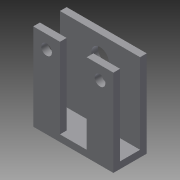
# Autodesk Inventor part: Speaker Mount
Saved by Autodesk Inventor 2014 SP2 (Build 180246200, 246)
## iProperties
Created: 2015-08-11
Part Number: Speaker Mount
Material: Generic
Document SubType Name: Modeling
Designer: Devon
Density: 1 g/cm^3
Appearance: Default
Author: Devon
Autodesk Inventor part; units mm, degrees
ref_plane "YZ Plane" through (0, 0, 0) normal (1, 0, 0) x (0, 1, 0)
ref_plane "XZ Plane" through (0, 0, 0) normal (0, 1, 0) x (-1, 0, 0)
ref_plane "XY Plane" through (0, 0, 0) normal (0, 0, 1) x (1, 0, 0)
sketch "Sketch1" plane through (0, 0, 0) normal (0, 0, 1) x (1, 0, 0)
  line L0 (-7.6264, 7.0378) -> (30.4736, 7.0378)
  line L1 (30.4736, 7.0378) -> (30.4736, -31.0622)
  line L2 (-7.6264, -31.0622) -> (-7.6264, 7.0378)
  circle A0 centre (11.4236, -2.4872) radius 4.1656
  circle A1 centre (11.4236, -21.5372) radius 4.1656
  line L3 (30.4736, -31.0622) -> (30.4736, -34.2372)
  line L4 (30.4736, -34.2372) -> (-7.6264, -34.2372)
  line L5 (-7.6264, -34.2372) -> (-7.6264, -31.0622)
  point P0 (0, 0)
  dimension "d0" = 38.1
  dimension "d1" = 38.1
  dimension "d4" = 8.3312
  dimension "d5" = 8.3312
  dimension "d8" = 3.175
  constraints: 12 end point, 2 centre point, 2 parallel, 2 perpendicular, 1 horizontal
  measures "d0" distance of L1.end L2.start
  measures "d1" distance of L0.end L1.end
  measures "d4" diameter of A0
  measures "d5" diameter of A1
  measures "d8" distance of L1.end L3.end
extrude "Extrusion1" add sketch "Sketch1" along normal blind 3.175
sketch "Sketch2" plane through (0, 0, 3.175) normal (0, 0, 1) x (1, 0, 0)
  line L0 (30.4736, -34.2372) -> (30.4736, 7.0378) projected
  line L1 (-7.6264, -34.2372) -> (30.4736, -34.2372)
  line L2 (30.4736, -34.2372) -> (30.4736, -31.0622)
  line L3 (30.4736, -31.0622) -> (-7.6264, -31.0622)
  line L4 (-7.6264, -31.0622) -> (-7.6264, -34.2372)
  point P0 (0, 0)
  dimension "d9" = 3.175
  constraints: 8 end point, 2 parallel, 1 horizontal, 1 perpendicular, 1 point on line
  measures "d9" distance of L2.end L1.end
extrude "Extrusion2" add sketch "Sketch2" along normal blind 12.7
sketch "Sketch3" plane through (-7.6264, -31.0622, 3.175) normal (0, 1, 0) x (1, 0, 0)
  line L0 (38.1, 0) -> (38.1, -12.7) projected
  line L1 (38.1, -12.7) -> (38.1, -9.525)
  line L2 (0, -9.525) -> (0, -12.7)
  line L3 (0, -9.525) -> (12.7, -9.525)
  line L4 (38.1, -9.525) -> (25.4, -9.525)
  line L5 (12.7, -9.525) -> (12.7, -12.7)
  line L6 (25.4, -9.525) -> (25.4, -12.7)
  line L7 (0, -12.7) -> (12.7, -12.7)
  line L8 (25.4, -12.7) -> (38.1, -12.7)
  point P0 (7.6264, 3.175)
  dimension "d12" = 3.175
  dimension "d13" = 12.7
  dimension "d14" = 12.7
  constraints: 16 end point, 5 perpendicular, 2 equal length, 2 horizontal, 1 point on line
  measures "d12" distance of L1.end L1.start
  measures "d13" distance of L2.start L3.end
  measures "d14" distance of L1.end L4.end
extrude "Extrusion3" add sketch "Sketch3" along normal blind 38.1
sketch "Sketch4" plane through (0, 0, 15.875) normal (0, 0, 1) x (1, 0, 0)
  line L0 (17.7736, 7.0378) -> (30.4736, 7.0378) projected
  line L1 (-7.6264, 7.0378) -> (5.0736, 7.0378) projected
  line L2 (-7.6264, -34.2372) -> (-7.6264, 7.0378) projected
  line L3 (-1.2764, 7.0378) -> (-1.2764, 0.6878)
  line L4 (24.1236, 7.0378) -> (24.1236, 0.6878)
  point P0 (0, 0)
  dimension "d17" = 6.35
  dimension "d18" = 6.35
  constraints: 4 end point, 2 midpoint, 2 parallel
  measures "d17" distance of L3.start L3.end
  measures "d18" distance of L4.start L4.end
hole "Hole1" at (-1.2764, 0.6878, 15.875) at (24.1236, 0.6878, 15.875) direction (0, 0, -1) diameter 5.08 depth 6.35 tip angle 118
body "Solid1"
